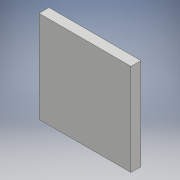
# Autodesk Inventor part: DiffusorCapThin
Saved by Autodesk Inventor 2018 (Build 220112000, 112)
## iProperties
Created: 2018-05-11
Part Number: DiffusorCapThin
Material: Generic
Document SubType Name: Modeling
Designer: a
Density: 1 g/cm^3
Appearance: Default
Author: a
## iProperties of the stored document DiffusorCap_3DPrint.ipt
Created: 2018-05-11
Part Number: DiffusorCap_3DPrint
Material: Generic
Document SubType Name: Modeling
Designer: a
Density: 1 g/cm^3
Appearance: Default
Author: a
Autodesk Inventor part; units mm, degrees
ref_plane "YZ Plane" through (0, 0, 0) normal (1, 0, 0) x (0, 1, 0)
ref_plane "XZ Plane" through (0, 0, 0) normal (0, 1, 0) x (-1, 0, 0)
ref_plane "XY Plane" through (0, 0, 0) normal (0, 0, 1) x (1, 0, 0)
sketch "Sketch1" plane through (0, 0, 0) normal (0, 1, 0) x (-1, 0, 0)
  line L0 (0, 0) -> (74, 0)
  line L1 (74, 0) -> (74, -74)
  line L2 (74, -74) -> (0, -74)
  line L3 (0, -74) -> (0, 0)
  dimension "d0" = 74
  dimension "d1" = 74
  constraints: 8 end point, 2 parallel, 1 horizontal, 1 perpendicular
  measures "d0" distance of L1.end L2.end
  measures "d1" distance of L0.end L1.end
extrude "Extrusion1" add sketch "Sketch1" along normal blind 10
sketch "Sketch2" plane through (0, 10, 0) normal (0, 1, 0) x (1, 0, 0)
  line L0 (0, 0) -> (0, 74) projected
  line L1 (0, 74) -> (-74, 74) projected
  line L2 (0, 0) -> (-74, 0)
  line L3 (-74, 0) -> (-74, 74)
  line L4 (-74, 74) -> (0, 74)
  line L5 (0, 74) -> (0, 0)
  line L6 (-72.5, 72.5) -> (-72.5, 1.5)
  line L7 (-72.5, 1.5) -> (-1.5, 1.5)
  line L8 (-1.5, 1.5) -> (-1.5, 72.5)
  line L9 (-1.5, 72.5) -> (-72.5, 72.5)
  dimension "d4" = 1.5
  constraints: 16 end point, 4 parallel, 2 perpendicular, 1 horizontal, 3 other
  measures "d4" distance between parallel lines of L3 L6
extrude "Extrusion2" add sketch "Sketch2" along normal blind 5
sketch "Sketch3" plane through (0, 0, 0) normal (0, -1, 0) x (1, 0, 0)
  line L0 (0, 0) -> (0, -74) projected
  line L1 (0, 0) -> (-74, 0)
  line L2 (-74, 0) -> (-74, -74)
  line L3 (-74, -74) -> (0, -74)
  line L4 (0, -74) -> (0, 0)
  constraints: 8 end point, 2 parallel, 1 horizontal, 1 perpendicular
extrude "Extrusion3" cut sketch "Sketch3" against normal blind 5
sketch "Sketch4" plane through (0, 5, 0) normal (0, -1, 0) x (1, 0, 0)
  line L0 (0, 0) -> (0, -74) projected
  line L1 (-74, -74) -> (0, -74)
  line L2 (0, -74) -> (0, 0)
  line L3 (0, 0) -> (-74, 0)
  line L4 (-74, 0) -> (-74, -74)
  constraints: 8 end point, 2 parallel, 1 horizontal, 1 perpendicular
extrude "Extrusion4" cut sketch "Sketch4" against normal blind 2
body "Solid1"
